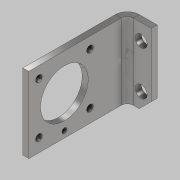
# Autodesk Inventor part: RR-PCSS-MSK
Saved by Autodesk Inventor 2021 (Build 250183000, 183)
## iProperties
Created: 2021-09-29
Part Number: RR-PCSS-MSK
Material: Stal nierdzewna
Document SubType Name: Konstrukcja blachowa
Designer: Marcin Sobczak
Density: 8 g/cm^3
Sheet Metal Rule: Domyślny_mm
Appearance: Częściowo polerowana
Flat Pattern Width: 3.8 cm
Flat Pattern Length: 6.22858 cm
Flat Pattern Area: 23.6686 cm^2
Sheet Metal Width: 38,000 mm
Sheet Metal Length: 62,286 mm
Sheet Metal Area: 2366,862 mm^2
Project: Ramie robotyczne
Description: Mocowanie silnika krokowego
Mass: 43.481 g
Surface Area: 47.0316 cm^2
Volume: 5.43512 cm^3
Author: marci
Autodesk Inventor part; units mm, degrees
ref_plane "YZ Plane" through (0, 0, 0) normal (1, 0, 0) x (0, 1, 0)
ref_plane "XZ Plane" through (0, 0, 0) normal (0, 1, 0) x (-1, 0, 0)
ref_plane "XY Plane" through (0, 0, 0) normal (0, 0, 1) x (1, 0, 0)
sketch "Szkic1" plane through (0, 0, 0) normal (1, 0, 0) x (0, 1, 0)
  line L0 (0, 0) -> (38, 0)
  line L1 (38, 0) -> (38, 52.5)
  line L2 (38, 52.5) -> (0, 52.5)
  line L3 (0, 52.5) -> (0, 0)
  circle A0 centre (19.5, 34.65) radius 12
  circle A1 centre (6.65, 47.5) radius 1.65
  circle A2 centre (32.35, 47.5) radius 1.65
  circle A3 centre (6.65, 21.8) radius 1.65
  circle A4 centre (32.35, 21.8) radius 1.65
  dimension "d0" = 38
  dimension "d1" = 52.5
  dimension "d2" = 24
  dimension "d3" = 17.85
  dimension "d5" = 3.3
  dimension "d6" = 3.3
  dimension "d7" = 3.3
  dimension "d8" = 3.3
  dimension "d9" = 25.7
  dimension "d10" = 25.7
  dimension "d11" = 25.7
  dimension "d12" = 25.7
  dimension "d13" = 5
  dimension "d14" = 5
  dimension "d15" = 12.85
  dimension "d16" = 12.85
  dimension "d38" = 18.5
  measures "d0" distance of L2.end L1.end
  measures "d1" distance of L1.end L0.end
  measures "d2" diameter of A0
  measures "d3" distance from line of L2 A0.centre
  measures "d5" diameter of A1
  measures "d6" diameter of A2
  measures "d7" diameter of A3
  measures "d8" diameter of A4
  measures "d9" distance of A4.centre A2.centre
  measures "d10" distance of A2.centre A1.centre
  measures "d11" distance of A3.centre A1.centre
  measures "d12" distance of A4.centre A3.centre
  measures "d13" distance from line of L2 A1.centre
  measures "d14" distance from line of L2 A2.centre
  measures "d15" horizontal distance of A0.centre A2.centre
  measures "d16" horizontal distance of A0.centre A4.centre
  measures "d38" distance from line of L1 A0.centre
extrude "Płyta1" add sketch "Szkic1" along normal blind 3
sketch "Szkic2" plane through (0, 38, 3) normal (0, 0, -1) x (-1, 0, 0)
  line L0 (0, -38) -> (0, 0)
  line L1 (0, 0) -> (-15, 0)
  line L2 (-15, 0) -> (-15, -38)
  line L3 (-15, -38) -> (0, -38)
  constraints: 6 end point, 1 horizontal, 1 perpendicular, 1 vertical
edge flange "Kołnierz1" height 15 angle 90 thickness 3 bend radius 3 thickness toward (0, 0, -1) relief straight relief width 3 relief depth 1.5 edges at (3, 19, 0) wall of the first edge with corners at (0, 0, 3) (0, 38, 3) (15, 38, 3) (15, 0, 3)
bend "Zagięcie1"
corner "Narożnik1"
sketch "Szkic3" plane through (15, 0, 3) normal (0, 0, 1) x (1, 0, 0)
  circle A0 centre (-5, 8) radius 3
  circle A1 centre (-5, 30) radius 3
  line L0 (-9, 38) -> (0, 38) projected
  line L1 (-9, 0) -> (0, 0) projected
  line L2 (0, 0) -> (0, 38) projected
  point P0 (-15, 0)
  dimension "d30" = 6
  dimension "d31" = 6
  dimension "d32" = 8
  dimension "d33" = 8
  dimension "d34" = 5
  dimension "d35" = 5
  constraints: 2 centre point
  measures "d30" diameter of A0
  measures "d31" diameter of A1
  measures "d32" distance from line of L0 A1.centre
  measures "d33" distance from line of L1 A0.centre
  measures "d34" distance from line of L2 A0.centre
  measures "d35" distance from line of L2 A1.centre
extrude "Wytnij1" cut sketch "Szkic3" against normal blind 3
chamfer "Fazowanie narożnika1" distance 6 angle 45 1 edges at (15, 0, 1.5)
sketch "Szkic4" plane through (3, 0, 0) normal (1, 0, 0) x (0, 0, -1)
  point P0 (-34.65, 3.2537)
hole "Otwór1" at (3, 3.2537, 34.65) direction (-1, 0, 0) diameter 2.459 depth 3.7451 tip angle 120 thread size "M3x0.5" class "6H" standard "ISO Metric profile"
equation "\"d36\" = Grubość"
equation "\"d19\" = Grubość"
equation "\"d20\" = SzerokośćGięciaPodcięcia"
equation "\"d21\" = GłębokośćGięciaPodcięcia"
equation "\"d22\" = MinimalnaPozostałość"
equation "\"d23\" = PromieńPrzejścia"
equation "\"d26\" = PromieńGięcia"
equation "\"d27\" = RozmiarPodcięciaNarożnika"
equation "\"d28\" = Wielk_odstępu"
equation "\"d29\" = Rozmiar_promienia_Jacobiego"
equation "\"PromieńGięcia\" = Grubość"
equation "\"SzerokośćGięciaPodcięcia\" = Grubość"
equation "\"GłębokośćGięciaPodcięcia\" = 0.5 * Grubość"
equation "\"RozmiarPodcięciaNarożnika\" = 4 * Grubość"
equation "\"MinimalnaPozostałość\" = 2 * Grubość"
equation "\"PromieńPrzejścia\" = PromieńGięcia"
equation "\"Rozmiar_promienia_Jacobiego\" = PromieńGięcia"
equation "\"Wielk_odstępu\" = Grubość"
equation "\"Grubość\" = 3"
